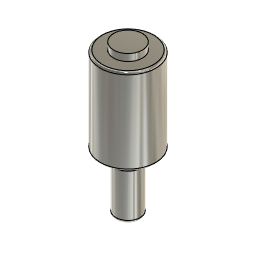
ERK-1 (Autodesk Fusion 360 archive; units mm, degrees)
design "Spindle 200W"
Autodesk Fusion 360 part; units mm, degrees
sketch "Sketch2" plane through (0, 0, 0) normal (0, 0, 1) x (1, 0, 0)
  circle A0 centre (0, 0) radius 26
  dimension "d9" = 52
  constraint coincident A0.centre origin
  measures "d9" diameter of A0
extrude "Extrude1" add sketch "Sketch2" along normal blind 80.5
sketch "Sketch3" plane through (0, 0, 80.5) normal (0, 0, 1) x (-1, 0, 0)
  circle A0 centre (0, 0) radius 26
  circle A1 centre (0, 0) radius 13.5
  dimension "d12" = 27
  constraint concentric A0 A1
  measures "d12" diameter of A1
extrude "Extrude2" add sketch "Sketch3" along normal blind 6.5 contours A1
sketch "Sketch4" plane through (0, 0, 0) normal (0, 0, -1) x (1, 0, 0)
  circle A0 centre (0, 0) radius 26
  circle A1 centre (0, 0) radius 13.5
  circle A2 centre (0, 17.5) radius 2
  circle A3 centre (-17.5, 0) radius 2
  circle A4 centre (0, -17.5) radius 2
  circle A5 centre (17.5, 0) radius 2
  dimension "d15" = 27
  dimension "d16" = 4
  dimension "d17" = 17.5
  dimension "d19" = 360
  constraint coincident A0.centre A1.centre
  constraint vertical A0.centre A2.centre
  measures "d15" diameter of A1
  measures "d16" diameter of A2
  measures "d17" vertical distance of A0.centre A2.centre
extrude "Extrude3" add sketch "Sketch4" along normal blind 6.5 contours A1
extrude "Extrude4" cut sketch "Sketch4" against normal blind 10 contours A2 | A3 | A4 | A5
sketch "Sketch5" plane through (0, 0, -6.5) normal (0, 0, -1) x (1, 0, 0)
  circle A0 centre (0, 0) radius 13.5
  circle A1 centre (0, 0) radius 6
  dimension "d25" = 12
  constraint concentric A0 A1
  measures "d25" diameter of A1
extrude "Extrude5" add sketch "Sketch5" along normal blind 3.5 contours A1
sketch "Sketch6" plane through (0, 0, -10) normal (0, 0, -1) x (1, 0, 0)
  circle A0 centre (0, 0) radius 6
  circle A1 centre (0, 0) radius 11.4801
  dimension "d30" = 22.9602
  constraint concentric A0 A1
  measures "d30" diameter of A1
extrude "Extrude6" add sketch "Sketch6" along normal blind 43 contours A0 | A1
fillet "Fillet1" radius 3 1 edges at (-10.7032, 4.1514, -53)
sketch "Sketch7" plane through (0, 0, -53) normal (0, 0, -1) x (1, 0, 0)
  circle A0 centre (0, 0) radius 8.4801
  circle A1 centre (0, 0) radius 3.5
  dimension "d35" = 7
  constraint concentric A0 A1
  measures "d35" diameter of A1
extrude "Extrude7" cut sketch "Sketch7" against normal blind 10 contours A1
fillet "Fillet2" radius 2 2 edges at (-24.2405, -9.402, 0) (-24.2405, -9.402, 80.5)
equation "diameter = 52 mm"
equation "nubDiameter = 27 mm"
equation "nubLength = 6.5 mm"
equation "motorLength = 80.5 mm"
equation "totalLength = 140 mm"
equation "colletLength = 43 mm"
equation "mountHoleDiameter = 4 mm"
equation "mountHoleDistanceFromAxle = ( 35 / 2 ) * 1 mm"
equation "d9 = diameter"
equation "d10 = motorLength"
equation "d12 = nubDiameter"
equation "d13 = nubLength"
equation "d15 = nubDiameter"
equation "d16 = mountHoleDiameter"
equation "d17 = mountHoleDistanceFromAxle"
equation "d20 = nubLength"
equation "axleDiameter = 12 mm"
equation "d25 = axleDiameter"
equation "d26 = axleLength"
equation "axleLength = totalLength - motorLength - nubLength * 2 - colletLength"
equation "colletDiameter = 22 mm"
equation "d31 = colletLength"

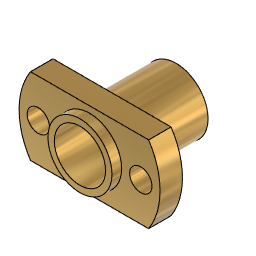
design "T8 Brass Nut"
Autodesk Fusion 360 part; units mm, degrees
sketch "Sketch1" plane through (0, 0, 0) normal (0, 1, 0) x (1, 0, 0)
  circle A0 centre (0, 0) radius 11
  circle A1 centre (0, 0) radius 5
  circle A2 centre (0, 0) radius 4
  line L0 (20, 6) -> (-20, 6)
  line L1 (-20, 6) -> (-20, -6) construction
  line L2 (-20, -6) -> (20, -6)
  line L3 (20, -6) -> (20, 6) construction
  line L4 (20, 6) -> (-20, -6) construction
  line L5 (-20, 6) -> (20, -6) construction
  circle A3 centre (8, 0) radius 1.75
  circle A4 centre (-8, 0) radius 1.75
  dimension "d11" = 22
  dimension "d12" = 10
  dimension "d13" = 8
  dimension "d14" = 40
  dimension "d15" = 12
  dimension "d22" = 3.5
  dimension "d23" = 3.5
  dimension "d24" = 8
  dimension "d25" = 8
  constraint coincident A0.centre A1.centre
  constraint concentric A0 A2
  constraint horizontal L0
  constraint perpendicular L0 L1
  constraint parallel L0 L2
  constraint parallel L1 L3
  constraint coincident L4 A0.centre
  constraint coincident L5 A0.centre
  constraint horizontal A0.centre A4.centre
  constraint horizontal A3.centre A4.centre
  measures "d11" diameter of A0
  measures "d12" diameter of A1
  measures "d13" diameter of A2
  measures "d14" distance of L1.end L2.end
  measures "d15" distance of L0.end L1.end
  measures "d22" diameter of A4
  measures "d23" diameter of A3
  measures "d24" distance of A0.centre A3.centre
  measures "d25" distance of A0.centre A4.centre
extrude "Extrude1" add sketch "Sketch1" along normal blind 3.5 contours A0 L0 L2 | A1 | A3 | A4
extrude "Extrude2" add sketch "Sketch1" against normal blind 1.5 contours A1
extrude "Extrude3" add sketch "Sketch1" along normal blind 13.5 contours A1
extrude "Extrude4" cut sketch "Sketch1" along normal blind 3.5 contours A3 | A4
equation "fullLength = 15 mm"
equation "flangeThickness = 3.5 mm"
equation "frontStickout = 1.5 mm"
equation "rearStickout = 10 mm"
equation "id = 8 mm"
equation "od = 10 mm"
equation "flangeHeight = 12 mm"
equation "flangeDiameter = 22 mm"
equation "screwHoleDiameter = 3.5 mm"
equation "screwHoleSpacing = 16 mm"
equation "d11 = flangeDiameter"
equation "d12 = od"
equation "d13 = id"
equation "d15 = flangeHeight"
equation "d16 = flangeThickness"
equation "d18 = -frontStickout"
equation "d20 = flangeThickness + rearStickout"
equation "d22 = screwHoleDiameter"
equation "d23 = screwHoleDiameter"
equation "d24 = screwHoleSpacing / 2"
equation "d25 = d24"
equation "d26 = flangeThickness"

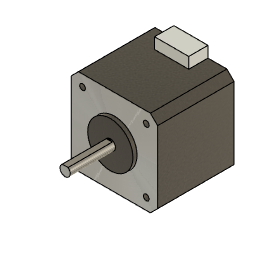
design "NEMA 17 37mm"
Autodesk Fusion 360 part; units mm, degrees
sketch "Sketch1" plane through (0, 0, 0) normal (0, 1, 0) x (1, 0, 0)
  line L0 (21, 21) -> (-21, 21)
  line L1 (-21, 21) -> (-21, -21)
  line L2 (-21, -21) -> (21, -21)
  line L3 (21, -21) -> (21, 21)
  line L4 (21, 21) -> (-21, -21) construction
  line L5 (-21, 21) -> (21, -21) construction
  circle A0 centre (0, 0) radius 11
  circle A1 centre (0, 0) radius 2.5
  circle A2 centre (-15.5, -15.5) radius 1.4
  circle A3 centre (15.5, -15.5) radius 1.4
  circle A4 centre (15.5, 15.5) radius 1.4
  circle A5 centre (-15.5, 15.5) radius 1.4
  dimension "d16" = 42
  dimension "d17" = 42
  dimension "d20" = 22
  dimension "d21" = 5
  dimension "d22" = 2.8
  dimension "d23" = 15.5
  dimension "d25" = 360
  constraint horizontal L0
  constraint perpendicular L0 L1
  constraint parallel L0 L2
  constraint parallel L1 L3
  constraint coincident L4 A0.centre
  constraint coincident L5 A0.centre
  constraint coincident A0.centre A1.centre
  constraint concentric A0 A1
  constraint coincident L4 A2.centre
  measures "d16" distance of L1.end L2.end
  measures "d17" distance of L0.end L1.end
  measures "d20" diameter of A0
  measures "d21" diameter of A1
  measures "d22" diameter of A2
  measures "d23" horizontal distance of A0.centre A2.centre
extrude "Extrude1" add sketch "Sketch1" along normal blind 37.2 contours L0 L1 L2 L3 | A0 | A1 | A2 | A3 | A4 | A5 makes body 1
extrude "Extrude2" cut sketch "Sketch1" along normal blind 4.5 contours A2 | A3 | A4 | A5 bodies 1
extrude "Extrude3" add sketch "Sketch1" against normal blind 2 contours A0 bodies 1
extrude "Extrude4" add sketch "Sketch1" against normal blind 24 separate body contours A1 makes body 2
sketch "Sketch2" plane through (0, 37.2, 0) normal (0, 1, 0) x (-1, 0, 0)
  line L0 (-21, 21) -> (-21, -21)
  line L1 (-21, -21) -> (21, -21)
  line L2 (21, -21) -> (21, 21)
  line L3 (21, 21) -> (-21, 21)
  circle A0 centre (0, 0) radius 4.575
  dimension "d32" = 9.15
  constraint coincident A0.centre origin
  measures "d32" diameter of A0
extrude "Extrude5" cut sketch "Sketch2" against normal blind 3.41 contours A0 bodies 1
sketch "Sketch3" plane through (0, -24, 0) normal (0, -1, 0) x (1, 0, 0)
  circle A0 centre (0, 0) radius 2.5
  line L0 (-1.4309, 2.05) -> (1.4309, 2.05)
  dimension "d35" = 2.05
  constraint coincident A0 L0.start
  constraint coincident A0 L0.end
  constraint horizontal L0
  measures "d35" distance of A0.centre L0
extrude "Extrude6" cut sketch "Sketch3" against normal blind 21.5 contours A0 L0 picked at (-0.0715, 2.241) bodies 2
chamfer "Chamfer1" distance 3.5 angle 45 4 edges at (21, 18.6, 21) (21, 18.6, -21) (-21, 18.6, 21) (-21, 18.6, -21) on bodies 1
sketch "Sketch4" plane through (0, 0, 21) normal (0, 0, 1) x (-1, 0, 0)
  line L0 (17.5, -37.2) -> (17.5, 0)
  line L1 (17.5, 0) -> (-17.5, 0)
  line L2 (-17.5, 0) -> (-17.5, -37.2)
  line L3 (-17.5, -37.2) -> (17.5, -37.2)
  line L4 (8.31, -37.2) -> (-8.31, -37.2)
  line L5 (-8.31, -37.2) -> (-8.31, -27.82)
  line L6 (-8.31, -27.82) -> (8.31, -27.82)
  line L7 (8.31, -27.82) -> (8.31, -37.2)
  point P0 (0, -37.2)
  point P1 (0, -37.2)
  dimension "d41" = 16.62
  dimension "d42" = 9.38
  constraint horizontal L4
  constraint vertical L5
  constraint horizontal L6
  constraint vertical L7
  constraint midpoint L4 P1
  constraint midpoint L3 P1
  constraint coincident P1 P0
  measures "d41" distance of L5.end L6.end
  measures "d42" distance of L4.end L5.end
extrude "Extrude7" add sketch "Sketch4" along normal blind 5.4 separate body contours L3 L4 L5 L6 L7 makes body 3
equation "length = 37.2 mm"
equation "width = 42 mm"
equation "nubDiameter = 22 mm"
equation "shaftDiameter = 5 mm"
equation "shaftDiameterAtFlat = 4.55 mm"
equation "shaftLength = 24 mm"
equation "nubHeight = 2 mm"
equation "connectorWidth = 16.62 mm"
equation "connectorHeight = 9.38 mm"
equation "connectorLength = 5.4 mm"
equation "screwHole = 2.8 mm"
equation "rearHoleDiameter = 9.15 mm"
equation "rearHoleDepth = 3.41 mm"
equation "screwHoleSpacing = 31 mm"
equation "screwHoleDepth = 4.5 mm"
equation "d16 = width"
equation "d17 = width"
equation "d18 = length"
equation "d20 = nubDiameter"
equation "d21 = shaftDiameter"
equation "d22 = screwHole"
equation "d23 = screwHoleSpacing / 2"
equation "d26 = screwHoleDepth"
equation "d28 = -nubHeight"
equation "d30 = -shaftLength"
equation "d32 = rearHoleDiameter"
equation "d33 = -rearHoleDepth"
equation "d35 = shaftDiameter / 2 - ( shaftDiameter - shaftDiameterAtFlat )"
equation "shaftFlatLength = 21.5 mm"
equation "d37 = -shaftFlatLength"
equation "chamfer = 3.5 mm"
equation "d40 = chamfer"
equation "d41 = connectorWidth"
equation "d42 = connectorHeight"
equation "d43 = connectorLength"
named bodies: "Body", "Shaft", "Connector"

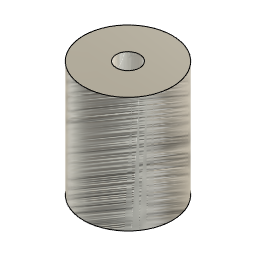
design "Flexible Coupling"
Autodesk Fusion 360 part; units mm, degrees
sketch "Sketch1" plane through (0, 0, 0) normal (0, 0, 1) x (1, 0, 0)
  circle A0 centre (0, 0) radius 9.5
  circle A1 centre (0, 0) radius 4
  dimension "d3" = 19
  dimension "d6" = 8
  constraint coincident A0.centre A1.centre
  constraint concentric A0 A1
  measures "d3" diameter of A0
  measures "d6" diameter of A1
extrude "Extrude1" add sketch "Sketch1" along normal blind 24.8 contours A0 | A1
sketch "Sketch2" plane through (0, 0, 24.8) normal (0, 0, 1) x (-1, 0, 0)
  circle A0 centre (0, 0) radius 9.5
  circle A1 centre (0, 0) radius 2.5
  dimension "d7" = 5
  constraint concentric A0 A1
  measures "d7" diameter of A1
extrude "Extrude2" cut sketch "Sketch2" against normal blind 24.8 contours A1
extrude "Extrude3" cut sketch "Sketch1" along normal blind 12.4 contours A1
equation "length = 24.8 mm"
equation "diameter = 19 mm"
equation "d3 = diameter"
equation "d4 = length"
equation "d8 = -length"
equation "d10 = length / 2"

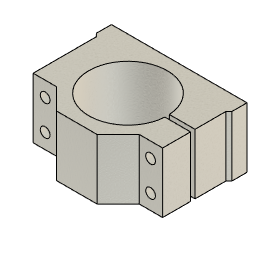
design "Spindle Clamp 52mm"
Autodesk Fusion 360 part; units mm, degrees
sketch "Sketch1" plane through (0, 0, 0) normal (0, 0, 1) x (1, 0, 0)
  circle A0 centre (0, -34) radius 26
  line L0 (-45, 0) -> (45, 0)
  line L1 (45, 0) -> (45, -10)
  line L2 (45, -10) -> (43, -10)
  line L3 (43, -10) -> (43, -54)
  line L4 (43, -54) -> (27.5, -54)
  line L5 (27.5, -54) -> (13.5, -68)
  line L6 (13.5, -68) -> (-13.5, -68)
  line L7 (-13.5, -68) -> (-27.5, -54)
  line L8 (-27.5, -54) -> (-43, -54)
  line L9 (-43, -54) -> (-43, -10)
  line L10 (-43, -10) -> (-45, -10)
  line L11 (-45, -10) -> (-45, 0)
  line L12 (0, 0) -> (0, -68) construction
  line L13 (0, -32.5) -> (50.9949, -32.5)
  line L14 (50.9949, -32.5) -> (50.9949, -35.5)
  line L15 (50.9949, -35.5) -> (0, -35.5)
  line L16 (0, -35.5) -> (0, -32.5)
  point P0 (0, -34)
  dimension "d10" = 52
  dimension "d11" = 34
  dimension "d13" = 10
  dimension "d14" = 34
  dimension "d15" = 2
  dimension "d16" = 90
  dimension "d19" = 54
  dimension "d22" = 135
  dimension "d23" = 27
  dimension "d25" = 3
  constraint vertical L12.start A0.centre
  constraint horizontal L0
  constraint perpendicular L0 L1
  constraint perpendicular L1 L2
  constraint perpendicular L2 L3
  constraint perpendicular L3 L4
  constraint perpendicular L3 L6
  constraint parallel L6 L8
  constraint perpendicular L8 L9
  constraint perpendicular L9 L10
  constraint vertical L11
  constraint midpoint L0 L12.start
  constraint coincident L12.start origin
  constraint coincident L6 L12.end
  constraint perpendicular L6 L12
  constraint symmetric L2 L10 L12
  constraint symmetric L4 L8 L12
  constraint symmetric L5 L7 L12
  constraint horizontal L13
  constraint vertical L14
  constraint horizontal L15
  constraint vertical L16
  constraint midpoint L16 P0
  constraint coincident P0 A0.centre
  measures "d10" diameter of A0
  measures "d11" distance of L12.start A0.centre
  measures "d13" distance of L0.start L10.end
  measures "d14" distance of P0 L6
  measures "d15" distance of L9.end L10.end
  measures "d16" distance of L0.start L0.end
  measures "d19" distance of L0 L8
  measures "d22" angle of L7 L8
  measures "d23" distance of L5.end L6.end
  measures "d25" distance of L13.end L14.end
extrude "Extrude1" add sketch "Sketch1" along normal blind 40 contours A0 L0 L1 L2 L3 L4 L5 L6 L7 L8 L9 L10 L11 L13 L15
chamfer "Chamfer1" distance 2 angle 45 2 edges at (43, -10, 20) (-43, -10, 20)
sketch "Sketch2" plane through (0, -54, 0) normal (0, -1, 0) x (1, 0, 0)
  line L0 (27.5, 0) -> (43, 0)
  line L1 (43, 0) -> (43, 40)
  line L2 (43, 40) -> (27.5, 40)
  line L3 (27.5, 40) -> (27.5, 0)
  circle A0 centre (35, 30) radius 3.25
  circle A1 centre (35, 10) radius 3.25
  dimension "d29" = 6.5
  dimension "d31" = 6.5
  dimension "d32" = 10
  dimension "d33" = 10
  dimension "d34" = 35
  constraint vertical A0.centre A1.centre
  measures "d29" diameter of A0
  measures "d31" diameter of A1
  measures "d32" distance of L0 A1.centre
  measures "d33" distance of L2 A0.centre
  measures "d34" horizontal distance of origin A1.centre
extrude "Extrude2" cut sketch "Sketch2" against normal blind 60 contours A0 | A1
mirror "Mirror1" about plane through (0, 0, 0) normal (1, 0, 0) of "Extrude2"
equation "diameter = 52 mm"
equation "screwHoleXSpacing = 70 mm"
equation "screwHoleYSpacing = 20 mm"
equation "height = 40 mm"
equation "screwHoleInset = 10 mm"
equation "gap = 3 mm"
equation "width = 90 mm"
equation "inset = 2 mm" comment "The undefined inset"
equation "insetHeight = 10 mm" comment "How far into the part the inset starts"
equation "d10 = diameter"
equation "d11 = spindleHoleInset + diameter / 2"
equation "spindleHoleInset = 8 mm"
equation "d13 = insetHeight"
equation "d14 = spindleHoleInset + diameter / 2"
equation "d15 = inset"
equation "d16 = width"
equation "length = 68 mm"
equation "lengthOfSolidPart = 54 mm" comment "this name sucks"
equation "d19 = lengthOfSolidPart"
equation "widthOfFrontFace = 27 mm"
equation "widthBeforeFrontAngle = 55 mm"
equation "d22 = 90 deg + 45 deg"
equation "d23 = widthOfFrontFace"
equation "d26 = height"
equation "d28 = inset"
equation "d29 = holeDiameter"
equation "holeDiameter = 6.5 mm"
equation "d31 = holeDiameter"
equation "d32 = screwHoleInset"
equation "d33 = screwHoleInset"
equation "d34 = screwHoleXSpacing / 2"

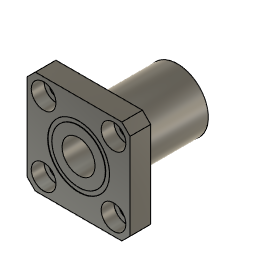
design "LMK8UU"
Autodesk Fusion 360 part; units mm, degrees
sketch "Sketch1" plane through (0, 0, 0) normal (0, 1, 0) x (1, 0, 0)
  circle A0 centre (0, 0) radius 4
  circle A1 centre (0, 0) radius 7.5
  line L0 (12.5, 12.5) -> (-12.5, 12.5)
  line L1 (-12.5, 12.5) -> (-12.5, -12.5)
  line L2 (-12.5, -12.5) -> (12.5, -12.5)
  line L3 (12.5, -12.5) -> (12.5, 12.5)
  line L4 (12.5, 12.5) -> (-12.5, -12.5) construction
  line L5 (-12.5, 12.5) -> (12.5, -12.5) construction
  circle A2 centre (-8.4853, -8.4853) radius 3
  circle A3 centre (-8.4853, -8.4853) radius 1.75
  circle A4 centre (0, 0) radius 6.5
  dimension "d8" = 8
  dimension "d9" = 15
  dimension "d10" = 25
  dimension "d11" = 25
  dimension "d14" = 6
  dimension "d15" = 12
  dimension "d16" = 3.5
  dimension "d28" = -1
  constraint coincident A0.centre A1.centre
  constraint concentric A0 A1
  constraint horizontal L0
  constraint perpendicular L0 L1
  constraint parallel L0 L2
  constraint parallel L1 L3
  constraint coincident L4 A0.centre
  constraint coincident L5 A0.centre
  constraint coincident L4 A2.centre
  constraint concentric A2 A3
  measures "d8" diameter of A0
  measures "d9" diameter of A1
  measures "d10" distance of L1.end L2.end
  measures "d11" distance of L0.end L1.end
  measures "d14" diameter of A2
  measures "d15" distance of A0.centre A2.centre
  measures "d16" diameter of A3
extrude "Extrude1" add sketch "Sketch1" along normal blind 5 contours A1 | L0 L1 L2 L3 | A2 | A3 | A4
extrude "Extrude3" add sketch "Sketch1" along normal blind 24 contours A1 | A4
extrude "Extrude2" cut sketch "Sketch1" along normal blind 3.1 contours A2 | A3
extrude "Extrude4" cut sketch "Sketch1" along normal blind 5 contours A3
pattern_circular "C-Pattern1" count 4 over 360 about axis through (0, 1.75, 0) along (0, 1, 0) of "Extrude2", "Extrude4"
chamfer "Chamfer1" distance 2 angle 45 4 edges at (12.5, 2.5, 12.5) (12.5, 2.5, -12.5) (-12.5, 2.5, 12.5) (-12.5, 2.5, -12.5)
extrude "Extrude5" cut sketch "Sketch1" along normal blind 0.1 contours A1
equation "od = 15 mm"
equation "id = 8 mm"
equation "length = 24 mm"
equation "flangeWidth = 25 mm"
equation "flangeThickness = 5 mm"
equation "screwHoleDiameter = 3.5 mm"
equation "screwHolesAtDiameter = 24 mm"
equation "d8 = id"
equation "d9 = od"
equation "d10 = flangeWidth"
equation "d11 = flangeWidth"
equation "screwHeadDiameter = 6 mm"
equation "screwHeadHeight = 3.1 mm"
equation "d14 = screwHeadDiameter"
equation "d15 = screwHolesAtDiameter / 2"
equation "d16 = screwHoleDiameter"
equation "d17 = flangeThickness"
equation "d19 = screwHeadHeight"
equation "d21 = length"
equation "d23 = flangeThickness"
